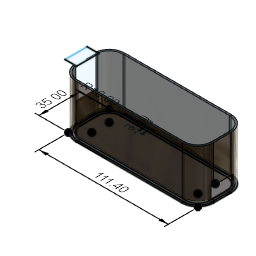
Body Bottom v11 (Autodesk Fusion 360 design; units mm, degrees)
Autodesk Fusion 360 part; units mm, degrees
sketch "Sketch1" plane through (0, 0, 0) normal (0, 0, 1) x (1, 0, 0)
  line L0 (10, 0) -> (101.4, 0)
  line L1 (111.4, 10) -> (111.4, 25)
  line L2 (101.4, 35) -> (10, 35)
  line L3 (0, 25) -> (0, 10)
  arc A0 (10, 35) -> (0, 25) centre (10, 25) ccw
  arc A1 (0, 10) -> (10, 0) centre (10, 10) ccw
  arc A2 (101.4, 0) -> (111.4, 10) centre (101.4, 10) ccw
  arc A3 (111.4, 25) -> (101.4, 35) centre (101.4, 25) ccw
  line L4 (-2, 25) -> (-2, 10)
  arc A4 (-2, 10) -> (10, -2) centre (10, 10) ccw
  line L5 (10, -2) -> (101.4, -2)
  arc A5 (101.4, -2) -> (113.4, 10) centre (101.4, 10) ccw
  line L6 (113.4, 10) -> (113.4, 25)
  arc A6 (113.4, 25) -> (101.4, 37) centre (101.4, 25) ccw
  line L7 (101.4, 37) -> (10, 37)
  arc A7 (10, 37) -> (-2, 25) centre (10, 25) ccw
  line L8 (-3.5, 25) -> (-3.5, 10)
  arc A8 (-3.5, 10) -> (10, -3.5) centre (10, 10) ccw
  line L9 (10, -3.5) -> (101.4, -3.5)
  arc A9 (101.4, -3.5) -> (114.9, 10) centre (101.4, 10) ccw
  line L10 (114.9, 10) -> (114.9, 25)
  arc A10 (114.9, 25) -> (101.4, 38.5) centre (101.4, 25) ccw
  line L11 (101.4, 38.5) -> (10, 38.5)
  arc A11 (10, 38.5) -> (-3.5, 25) centre (10, 25) ccw
  point P0 (111.4, 0)
  point P1 (0, 35)
  dimension "d1" = 111.4
  dimension "d2" = 35
  dimension "d3" = 10
  dimension "d4" = 2
  dimension "d5" = 3.5
  constraint horizontal L0
  constraint vertical L1
  constraint horizontal L2
  constraint vertical L3
  constraint coincident P1 L2
  constraint coincident P1 L3
  constraint tangent L2 A0
  constraint tangent L3 A0
  constraint coincident origin L0
  constraint coincident origin L3
  constraint tangent L0 A1
  constraint tangent L3 A1
  constraint equal A0 A1
  constraint coincident P0 L0
  constraint coincident P0 L1
  constraint tangent L0 A2
  constraint tangent L1 A2
  constraint equal A0 A2
  constraint tangent L1 A3
  constraint tangent L2 A3
  constraint equal A0 A3
  measures "d1" distance of origin P0
  measures "d2" distance of origin P1
  measures "d3" radius of A0
  measures "d12" distance of origin
extrude "Extrude1" add sketch "Sketch1" along normal blind 3 contours L0 L1 L2 L3 A0 A1 A2 A3 | L4 A4 L5 A5 L6 A6 L7 A7 | L8 A8 L9 A9 L10 A10 L11 A11
extrude "Extrude2" add sketch "Sketch1" along normal blind 45 contours L8 A8 L9 A9 L10 A10 L11 A11
sketch "Sketch2" plane through (0, 0, 45) normal (0, 0, 1) x (-1, 0, 0)
  arc A0 (-10, -37) -> (2, -25) centre (-10, -25) ccw
  line L0 (-10, -37) -> (-101.4, -37)
  arc A1 (-113.4, -25) -> (-101.4, -37) centre (-101.4, -25) ccw
  line L1 (-113.4, -25) -> (-113.4, -10)
  arc A2 (-101.4, 2) -> (-113.4, -10) centre (-101.4, -10) ccw
  line L2 (-101.4, 2) -> (-10, 2)
  arc A3 (2, -10) -> (-10, 2) centre (-10, -10) ccw
  line L3 (2, -10) -> (2, -25)
  arc A4 (-10, -38.5) -> (3.5, -25) centre (-10, -25) ccw
  line L4 (3.5, -25) -> (3.5, -10)
  arc A5 (3.5, -10) -> (-10, 3.5) centre (-10, -10) ccw
  line L5 (-10, 3.5) -> (-101.4, 3.5)
  arc A6 (-101.4, 3.5) -> (-114.9, -10) centre (-101.4, -10) ccw
  line L6 (-114.9, -10) -> (-114.9, -25)
  arc A7 (-114.9, -25) -> (-101.4, -38.5) centre (-101.4, -25) ccw
  line L7 (-101.4, -38.5) -> (-10, -38.5)
  line L8 (2, -17.5) -> (2, -27) construction
  line L9 (2, -27) -> (1, -27) construction
  line L10 (1, -27) -> (11, -27)
  line L11 (11, -27) -> (11, -8)
  line L12 (11, -8) -> (1, -8)
  line L13 (1, -8) -> (1, -27)
  dimension "d12" = 9.5
  dimension "d13" = 1
  dimension "d14" = 19
  constraint midpoint L3 L8.start
  constraint parallel L3 L8
  constraint perpendicular L8 L9
  constraint horizontal L10
  constraint vertical L11
  constraint horizontal L12
  constraint vertical L13
  measures "d12" distance of L8.start L8.end
  measures "d13" distance of L8.end L9.end
  measures "d14" distance of L9.end L12.end
extrude "Extrude5" cut sketch "Sketch2" against normal blind 28 contours A0 A3 L3 L10 L12 L13 | A0 A3 L3 A4 L4 A5 L10 L12 | A4 L4 A5 L10 L11 L12
sketch "Sketch3" plane through (114.9, 0, 0) normal (1, 0, 0) x (0, 1, 0)
  line L0 (10, 0) -> (25, 0)
  line L1 (25, 0) -> (25, 45)
  line L2 (25, 45) -> (10, 45)
  line L3 (10, 45) -> (10, 0)
  line L4 (17.5, 0) -> (17.5, 3) construction
  line L5 (17.5, 3) -> (27, 3) construction
  line L6 (27, 3) -> (8, 3)
  line L7 (8, 3) -> (8, 13)
  line L8 (8, 13) -> (27, 13)
  line L9 (27, 13) -> (27, 3)
  dimension "d19" = 3
  dimension "d20" = 9.5
  dimension "d21" = 19
  dimension "d22" = 10
  constraint midpoint L0 L4.start
  constraint perpendicular L0 L4
  constraint perpendicular L1 L5
  constraint horizontal L6
  constraint vertical L7
  constraint horizontal L8
  constraint vertical L9
  measures "d19" distance of L4.start L4.end
  measures "d20" distance of L4.end L5.end
  measures "d21" distance of L5.end L6.end
  measures "d22" distance of L5.end L8.end
extrude "Extrude6" cut sketch "Sketch3" against normal blind 10 contours L3 L6 L7 L8 | L1 L3 L6 L8 | L1 L6 L8 L9
